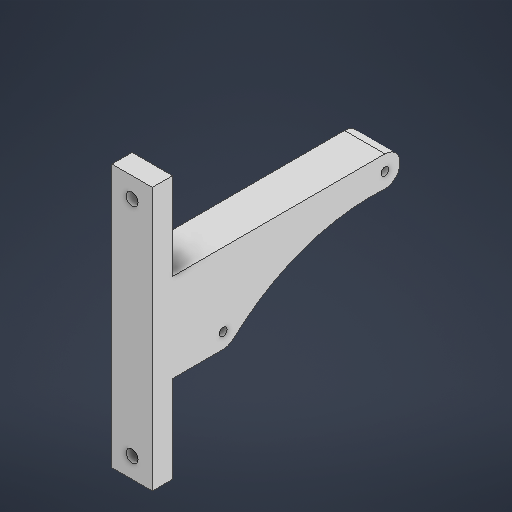
# Autodesk Inventor part: Caliper Bracket Mount
Saved by Autodesk Inventor 2026.1 (Build 301233000, 233)
## iProperties
Created: 2026-06-24
Part Number: Caliper Bracket Mount
Material: Generic
Document SubType Name: Modeling
Designer: share
Density: 1 g/cm^3
Appearance: Default
Author: share
Autodesk Inventor part; units mm, degrees
ref_plane "YZ Plane" through (0, 0, 0) normal (1, 0, 0) x (0, 1, 0)
ref_plane "XZ Plane" through (0, 0, 0) normal (0, 1, 0) x (-1, 0, 0)
ref_plane "XY Plane" through (0, 0, 0) normal (0, 0, 1) x (1, 0, 0)
sketch "Sketch1" plane through (0, 0, 0) normal (0, 0, 1) x (1, 0, 0)
  line L0 (-10, -65) -> (10, -65)
  line L1 (10, -65) -> (10, 65)
  line L2 (10, 65) -> (-10, 65)
  line L3 (-10, 65) -> (-10, -65)
  line L4 (-10, -65) -> (10, 65) construction
  line L5 (10, -65) -> (-10, 65) construction
  line L6 (0, 65) -> (0, -65) construction
  circle A0 centre (0, 55) radius 3
  circle A1 centre (0, -55) radius 3
  line L7 (10, 0) -> (-10, 0) construction
  point P0 (0, 0)
  dimension "d0" = 130
  dimension "d1" = 20
  dimension "d2" = 110
  dimension "d3" = 6
  constraints: 16 end point, 6 midpoint, 2 centre point, 2 parallel, 2 point on line, 1 horizontal, 1 perpendicular, 1 other
  measures "d0" distance between parallel lines of L0 L2
  measures "d1" distance between parallel lines of L1 L3
  measures "d2" distance of A1.centre A0.centre
  measures "d3" diameter of A0
extrude "Base" add sketch "Sketch1" against normal blind 10
sketch "Sketch7" plane through (0, 0, 0) normal (1, 0, 0) x (0, 0, -1)
  circle A0 centre (115, 14.3614) radius 2
  circle A1 centre (35, -14.3614) radius 2
  line L0 (115, 14.3614) -> (35, -14.3614) construction
  circle A2 centre (115, 14.3614) radius 7.5
  circle A3 centre (35, -14.3614) radius 7.5
  arc A4 (114.5372, 6.8757) -> (40.1186, -19.8432) centre (108.3665, -92.9337) ccw
  line L1 (-20, 0) -> (120, 0) construction
  line L2 (10, 65) -> (10, -65) projected
  line L3 (10, -21.8614) -> (122.5, -21.8614)
  line L4 (10, -65) -> (10, 65) projected
  line L5 (10, 21.8614) -> (122.5, 21.8614)
  line L6 (122.5, 21.8614) -> (122.5, -21.8614)
  line L7 (66.25, 21.8614) -> (66.25, -21.8614) construction
  line L8 (66.25, 0) -> (122.5, 0) construction
  line L9 (122.5, 21.8614) -> (10, 45.7099)
  line L10 (122.5, -21.8614) -> (10, -45.7099)
  point P0 (0, 0)
  point P1 (115, 21.8614)
  point P2 (35, -21.8614)
  dimension "d99" = 15
  dimension "d73" = 85
  dimension "d74" = 4
  dimension "d100" = 100
  dimension "d104" = 105
  dimension "d105" = 25
  dimension "d108" = 115
  constraints: 16 end point, 4 horizontal, 4 midpoint, 3 centre point, 3 point on line, 2 coincident, 2 point on circle, 1 collinear, 1 equal radius, 1 perpendicular, 1 symmetric about line, 1 vertical, 8 other
  measures "d73" distance of L0.start L0.end
  measures "d74" diameter of A0
  measures "d100" radius of A4
  measures "d104" distance from line of L0.start L2
  measures "d105" distance from line of L2 L0.end
  measures "d108" distance of L5.end L9.end
extrude "Extrusion13" add sketch "Sketch7" along normal mid plane 20 contours A2 | A4 A3 L3 L2 L5 A2 | A3
equation "\"d0\" = Main_Body_Height"
equation "\"d1\" = Main_Body_Width"
equation "\"d2\" = Upright_Hole_Spacing"
equation "\"Base_Thickness\" = 4"
equation "\"Main_Body_Height\" = 130"
equation "\"Main_Body_Width\" = 20"
equation "\"Upright_Hole_Spacing\" = 110"
body "Solid1"
